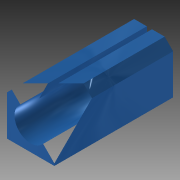
# Autodesk Inventor part: ZAxisCarriageRod
Saved by Autodesk Inventor 2015 (Build 190159000, 159)
## iProperties
Created: 2014-12-10
Part Number: ZAxisCarriageRod
Material: Generic
Document SubType Name: Modeling
Designer: Jack
Density: 1 g/cm^3
Appearance: Cyan
Author: Jack
Autodesk Inventor part; units mm, degrees
ref_plane "YZ Plane" through (0, 0, 0) normal (1, 0, 0) x (0, 1, 0)
ref_plane "XZ Plane" through (0, 0, 0) normal (0, 1, 0) x (-1, 0, 0)
ref_plane "XY Plane" through (0, 0, 0) normal (0, 0, 1) x (1, 0, 0)
sketch "Sketch1" plane through (0, 0, 0) normal (0, 1, 0) x (-1, 0, 0)
  arc A0 (-1.5, 9.3808) -> (1.5, 9.3808) centre (0, 0) ccw
  line L0 (14, -14) -> (14, 9.5)
  line L1 (14, 9.5) -> (9, 14.5)
  line L2 (9, 14.5) -> (1.5, 14.5)
  line L3 (1.5, 14.5) -> (1.5, 9.3808)
  line L4 (-1.5, 9.3808) -> (-1.5, 14.5)
  line L5 (-1.5, 14.5) -> (-9, 14.5)
  line L6 (-9, 14.5) -> (-14, 9.5)
  line L7 (-14, 9.5) -> (-14, -14)
  line L8 (14, -14) -> (-14, -14)
  dimension "d0" = 19
  dimension "d1" = 135
  dimension "d2" = 135
  dimension "d3" = 14
  dimension "d4" = 14
  dimension "d5" = 14.5
  dimension "d6" = 14
  dimension "d7" = 1.5
  dimension "d8" = 5
  constraints: 18 end point, 2 equal length, 2 parallel, 2 perpendicular, 2 point on circle, 2 point on line, 1 centre point, 1 coincident, 1 horizontal, 1 vertical
  measures "d0" diameter of A0
  measures "d1" angle of L0 L1
  measures "d2" angle of L7 L6
  measures "d3" distance from line of point (0, 0) L0
  measures "d4" distance from line of point (0, 0) L7
  measures "d5" distance from line of point (0, 0) L5
  measures "d6" distance from line of point (0, 0) L8
  measures "d7" distance from line of point (0, 0) L3
  measures "d8" horizontal distance of L6.end L5.end
extrude "Extrusion1" add sketch "Sketch1" along normal blind 70
body "Solid1"
